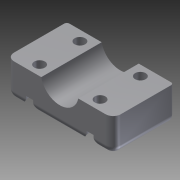
# Autodesk Inventor part: Z move plate
Saved by Autodesk Inventor 2012 (Build 160160000, 160)
## iProperties
Created: 2013-02-04
Part Number: Z move plate
Material: Default
Document SubType Name: Modeling
Designer: mce
Density: 1 g/cm^3
Author: mce
Autodesk Inventor part; units mm, degrees
ref_plane "YZ Plane" through (0, 0, 0) normal (1, 0, 0) x (0, 1, 0)
ref_plane "XZ Plane" through (0, 0, 0) normal (0, 1, 0) x (-1, 0, 0)
ref_plane "XY Plane" through (0, 0, 0) normal (0, 0, 1) x (1, 0, 0)
sketch "Sketch1" plane through (0, 0, 0) normal (0, 0, 1) x (1, 0, 0)
  line L0 (0, 0) -> (42.4, 0)
  line L1 (42.4, 0) -> (42.4, 24)
  line L2 (42.4, 24) -> (0, 24)
  line L3 (0, 24) -> (0, 0)
  circle A0 centre (9.2, 20) radius 2.1
  circle A1 centre (33.2, 20) radius 2.1
  circle A2 centre (33.2, 4) radius 2.1
  circle A3 centre (9.2, 4) radius 2.1
  dimension "d0" = 24
  dimension "d1" = 42.4
  dimension "d2" = 4.2
  dimension "d3" = 9.2
  dimension "d4" = 9.2
  dimension "d5" = 9.2
  dimension "d6" = 9.2
  dimension "d7" = 4
  dimension "d8" = 4
  dimension "d9" = 4
  dimension "d10" = 4
  constraints: 8 end point, 4 centre point, 3 equal radius, 2 horizontal, 2 vertical
  measures "d0" distance of L2.end L0.start
  measures "d1" distance of L0.start L0.end
  measures "d2" diameter of A0
  measures "d3" distance from line of L3 A0.centre
  measures "d4" distance from line of L3 A3.centre
  measures "d5" distance from line of L1 A2.centre
  measures "d6" distance from line of L1 A1.centre
  measures "d7" distance from line of L2 A0.centre
  measures "d8" distance from line of L0 A3.centre
  measures "d9" distance from line of L0 A2.centre
  measures "d10" distance from line of L2 A1.centre
extrude "Extrusion1" add sketch "Sketch1" along normal blind 13.5
sketch "Sketch2" plane through (0, 0, 0) normal (0, -1, 0) x (1, 0, 0)
  line L0 (42.4, 13.5) -> (0, 13.5) projected
  line L1 (0, 0) -> (0, 13.5) projected
  circle A0 centre (21.2, 15) radius 7.5
  dimension "d13" = 15
  dimension "d14" = 21.2
  dimension "d15" = 1.5
  constraints: 1 centre point
  measures "d13" diameter of A0
  measures "d14" distance from line of L1 A0.centre
  measures "d15" distance from line of A0.centre L0
extrude "Extrusion2" cut sketch "Sketch2" against normal through all
fillet "Fillet1" radius 3 3 edges at (42.4, 0, 6.75) (0, 0, 6.75) (21.2, 0, 0)
sketch "Sketch3" plane through (0, 0, 0) normal (0, 0, -1) x (-1, 0, 0)
  arc A0 (-31.3534, 3) -> (-35.0466, 3) centre (-33.2, 4) ccw projected
  arc A1 (-7.3534, 3) -> (-11.0466, 3) centre (-9.2, 4) ccw projected
  circle A2 centre (-33.2, 20) radius 2.1 projected
  circle A3 centre (-9.2, 20) radius 2.1 projected
  circle A4 centre (-33.2, 20) radius 4.25
  circle A5 centre (-9.2, 20) radius 4.25
  circle A6 centre (-9.2, 4) radius 4.25
  circle A7 centre (-33.2, 4) radius 4.25
  point P0 (0, 0)
  dimension "d20" = 8.5
  constraints: 4 centre point, 4 coincident, 3 equal radius
  measures "d20" diameter of A4
extrude "Extrusion3" cut sketch "Sketch3" against normal blind 4
sketch "Sketch4" plane through (21.2, 0, 15) normal (0, -1, 0) x (1, 0, 0)
  line L0 (-26.3081, 1.9971) -> (24.247, 1.9971)
  line L1 (24.247, 1.9971) -> (24.247, -18.7305)
  line L2 (24.247, -18.7305) -> (-26.3081, -18.7305)
  line L3 (-26.3081, -18.7305) -> (-26.3081, 1.9971)
  point P0 (-21.2, -15)
  constraints: 8 end point
extrude "Extrusion4" [suppressed]
fillet "Fillet3" radius 3 2 edges at (42.4, 13.5, 0) (0, 13.5, 0)
fillet "Fillet4" radius 1 7 edges at (41.5213, 24, 0.8787) (37.0181, 24, 0) (42.4, 24, 8.25) (21.2, 24, 0) (0.8787, 24, 0.8787) (0, 24, 8.25) (5.3819, 24, 0)
body "Solid1"
